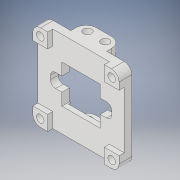
# Autodesk Inventor part: Camera_Cover
Saved by Autodesk Inventor 2019 (Build 230136000, 136)
## iProperties
Created: 2021-07-29
Part Number: Camera_Cover
Material: LCP 플라스틱
Document SubType Name: Modeling
Designer: user
Density: 1.626 g/cm^3
Appearance: 매끄러움 - 흰색
Mass: 4.96466 g
Surface Area: 31.5343 cm^2
Volume: 3.0533 cm^3
Author: user
Autodesk Inventor part; units mm, degrees
ref_plane "YZ Plane" through (0, 0, 0) normal (1, 0, 0) x (0, 1, 0)
ref_plane "XZ Plane" through (0, 0, 0) normal (0, 1, 0) x (-1, 0, 0)
ref_plane "XY Plane" through (0, 0, 0) normal (0, 0, 1) x (1, 0, 0)
sketch "스케치1" plane through (0, 0, 0) normal (0, 0, 1) x (1, 0, 0)
  line L0 (-16.9, 16.9) -> (16.9, 16.9)
  line L1 (16.9, 16.9) -> (16.9, -16.9)
  line L2 (16.9, -16.9) -> (-16.9, -16.9)
  line L3 (-16.9, -16.9) -> (-16.9, 16.9)
  point P0 (0, 0)
  dimension "d0" = 33.8
  dimension "d1" = 33.8
  dimension "d2" = 16.9
  dimension "d3" = 16.9
  constraints: 8 end point, 2 parallel, 1 horizontal, 1 perpendicular
  measures "d0" distance of L1.end L2.end
  measures "d1" distance of L0.end L1.end
  measures "d2" distance from line of L3 point (0, 0)
  measures "d3" distance from line of point (0, 0) L0
extrude "돌출1" add sketch "스케치1" along normal blind 3
sketch "스케치2" plane through (0, 0, 3) normal (0, 0, 1) x (1, 0, 0)
  circle A0 centre (-14, 14) radius 1.25
  circle A1 centre (14, 14) radius 1.25
  circle A2 centre (-14, -14) radius 1.25
  circle A3 centre (14, -14) radius 1.25
  line L0 (-16.9, 16.9) -> (-16.9, -16.9) projected
  line L1 (16.9, 16.9) -> (-16.9, 16.9) projected
  line L2 (16.9, -16.9) -> (16.9, 16.9) projected
  line L3 (-16.9, -16.9) -> (16.9, -16.9) projected
  line L4 (-16.9, 16.9) -> (-11.1, 16.9)
  line L5 (-11.1, 16.9) -> (-11.1, 11.1)
  line L6 (-11.1, 11.1) -> (-16.9, 11.1)
  line L7 (-16.9, 11.1) -> (-16.9, 16.9)
  line L8 (16.9, 16.9) -> (11.1, 16.9)
  line L9 (11.1, 16.9) -> (11.1, 11.1)
  line L10 (11.1, 11.1) -> (16.9, 11.1)
  line L11 (16.9, 11.1) -> (16.9, 16.9)
  line L12 (-16.9, -16.9) -> (-11.1, -16.9)
  line L13 (-11.1, -16.9) -> (-11.1, -11.1)
  line L14 (-11.1, -11.1) -> (-16.9, -11.1)
  line L15 (-16.9, -11.1) -> (-16.9, -16.9)
  line L16 (16.9, -16.9) -> (11.1, -16.9)
  line L17 (11.1, -16.9) -> (11.1, -11.1)
  line L18 (11.1, -11.1) -> (16.9, -11.1)
  line L19 (16.9, -11.1) -> (16.9, -16.9)
  point P0 (0, 0)
  dimension "d6" = 2.5
  dimension "d7" = 2.5
  dimension "d8" = 2.5
  dimension "d9" = 2.5
  dimension "d10" = 2.9
  dimension "d11" = 2.9
  dimension "d12" = 2.9
  dimension "d13" = 2.9
  dimension "d14" = 2.9
  dimension "d15" = 2.9
  dimension "d16" = 2.9
  dimension "d17" = 2.9
  dimension "d18" = 5.8
  dimension "d19" = 5.8
  dimension "d20" = 11.1
  dimension "d21" = 5.8
  dimension "d22" = 5.8
  dimension "d23" = 5.8
  dimension "d24" = 5.8
  dimension "d25" = 5.8
  dimension "d26" = 5.8
  constraints: 32 end point, 8 parallel, 4 centre point, 4 horizontal, 4 perpendicular
  measures "d6" diameter of A0
  measures "d7" diameter of A1
  measures "d8" diameter of A2
  measures "d9" diameter of A3
  measures "d10" distance from line of L0 A0.centre
  measures "d11" distance from line of L1 A0.centre
  measures "d12" distance from line of L2 A1.centre
  measures "d13" distance from line of L1 A1.centre
  measures "d14" distance from line of L3 A2.centre
  measures "d15" distance from line of L0 A2.centre
  measures "d16" distance from line of L3 A3.centre
  measures "d17" distance from line of L2 A3.centre
  measures "d18" distance of L5.end L6.end
  measures "d19" distance of L4.end L5.end
  measures "d20" distance from line of point (0, 0) L5
  measures "d21" distance of L10.end L9.end
  measures "d22" distance of L9.end L8.end
  measures "d23" distance of L14.end L13.end
  measures "d24" distance of L13.end L12.end
  measures "d25" distance of L17.end L18.end
  measures "d26" distance of L16.end L17.end
extrude "돌출2" add sketch "스케치2" along normal blind 2 contours A0 | A1 | A2 | A3 | L1 L5 L6 L0 | L14 L13 L3 L0 | L1 L2 L10 L9 | L17 L18 L2 L3
sketch "스케치3" plane through (0, 0, 5) normal (0, 0, 1) x (1, 0, 0)
  circle A0 centre (-14, 14) radius 1.5
  circle A1 centre (14, 14) radius 1.5
  circle A2 centre (14, -14) radius 1.5
  circle A3 centre (-14, -14) radius 1.5
  line L0 (-16.9, -11.1) -> (-16.9, -16.9) projected
  line L1 (-16.9, -16.9) -> (-11.1, -16.9) projected
  line L2 (11.1, -16.9) -> (16.9, -16.9) projected
  line L3 (16.9, -16.9) -> (16.9, -11.1) projected
  line L4 (11.1, 11.1) -> (16.9, 11.1) projected
  line L5 (16.9, 11.1) -> (16.9, 16.9) projected
  line L6 (-16.9, 16.9) -> (-16.9, 11.1) projected
  line L7 (-11.1, 16.9) -> (-16.9, 16.9) projected
  point P0 (0, 0)
  dimension "d29" = 3
  dimension "d30" = 3
  dimension "d31" = 3
  dimension "d32" = 3
  dimension "d33" = 2.9
  dimension "d34" = 2.9
  dimension "d35" = 2.9
  dimension "d36" = 2.9
  dimension "d37" = 2.9
  dimension "d38" = 2.9
  dimension "d39" = 2.9
  dimension "d40" = 2.9
  constraints: 4 centre point
  measures "d29" diameter of A0
  measures "d30" diameter of A1
  measures "d31" diameter of A2
  measures "d32" diameter of A3
  measures "d33" distance from line of L0 A3.centre
  measures "d34" distance from line of L1 A3.centre
  measures "d35" distance from line of L2 A2.centre
  measures "d36" distance from line of L3 A2.centre
  measures "d37" distance from line of L4 A1.centre
  measures "d38" distance from line of L5 A1.centre
  measures "d39" distance from line of L6 A0.centre
  measures "d40" distance from line of L7 A0.centre
extrude "돌출3" cut sketch "스케치3" against normal up to surface (5 mm away)
sketch "스케치4" plane through (0, 0, 3) normal (0, 0, 1) x (1, 0, 0)
  line L0 (-7.5, 7.5) -> (7.5, 7.5)
  line L1 (7.5, 7.5) -> (7.5, -7.5)
  line L2 (7.5, -7.5) -> (-7.5, -7.5)
  line L3 (-7.5, -7.5) -> (-7.5, 7.5)
  point P0 (0, 0)
  dimension "d43" = 15
  dimension "d44" = 15
  dimension "d45" = 7.5
  dimension "d46" = 7.5
  constraints: 8 end point, 2 parallel, 1 horizontal, 1 perpendicular
  measures "d43" distance of L1.end L2.end
  measures "d44" distance of L0.end L1.end
  measures "d45" distance from line of point (0, 0) L0
  measures "d46" distance from line of L3 point (0, 0)
extrude "돌출4" cut sketch "스케치4" against normal up to surface (3 mm away)
sketch "스케치5" plane through (0, 0, 3) normal (0, 0, 1) x (1, 0, 0)
  line L0 (-7.5, -2.75) -> (-12, -2.75)
  line L1 (-12, -2.75) -> (-12, 2.75)
  line L2 (-12, 2.75) -> (-7.5, 2.75)
  line L3 (-7.5, 2.75) -> (-7.5, -2.75)
  line L4 (7.5, 2.75) -> (12, 2.75)
  line L5 (12, 2.75) -> (12, -2.75)
  line L6 (12, -2.75) -> (7.5, -2.75)
  line L7 (7.5, -2.75) -> (7.5, 2.75)
  line L8 (-7.5, -7.5) -> (-7.5, 7.5) projected
  line L9 (7.5, 7.5) -> (7.5, -7.5) projected
  point P0 (0, 0)
  dimension "d49" = 4.5
  dimension "d50" = 5.5
  dimension "d51" = 4.5
  dimension "d52" = 5.5
  dimension "d53" = 0
  dimension "d54" = 2.75
  dimension "d55" = 0
  dimension "d56" = 2.75
  constraints: 16 end point, 4 parallel, 2 horizontal, 2 perpendicular
  measures "d49" distance of L1.end L2.end
  measures "d50" distance of L0.end L1.end
  measures "d51" distance of L5.end L6.end
  measures "d52" distance of L4.end L5.end
  measures "d53" distance between parallel lines of L8 L3
  measures "d54" distance from line of point (0, 0) L0
  measures "d55" distance between parallel lines of L9 L7
  measures "d56" distance from line of point (0, 0) L6
extrude "돌출5" cut sketch "스케치5" against normal up to surface (3 mm away)
fillet "모깎기1" radius 2 4 edges at (-12, 2.75, 1.5) (-12, -2.75, 1.5) (12, -2.75, 1.5) (12, 2.75, 1.5)
sketch "스케치6" plane through (0, 0, 0) normal (0, 0, -1) x (-1, 0, 0)
  line L0 (16.9, 16.9) -> (-16.9, 16.9) projected
  line L1 (-7, 16.9) -> (7, 16.9)
  line L2 (7, 16.9) -> (7, 12.9)
  line L3 (7, 12.9) -> (-7, 12.9)
  line L4 (-7, 12.9) -> (-7, 16.9)
  line L5 (-7, -16.9) -> (7, -16.9)
  line L6 (7, -16.9) -> (7, -12.9)
  line L7 (7, -12.9) -> (-7, -12.9)
  line L8 (-7, -12.9) -> (-7, -16.9)
  line L9 (-16.9, -16.9) -> (16.9, -16.9) projected
  point P0 (0, 0)
  dimension "d60" = 4
  dimension "d61" = 4
  dimension "d62" = 4
  dimension "d63" = 14
  dimension "d64" = 7
  dimension "d65" = 7
  dimension "d66" = 14
  constraints: 16 end point, 4 parallel, 2 horizontal, 2 perpendicular, 1 point on line
  measures "d60" distance between parallel lines of L7 L5
  measures "d61" distance between parallel lines of L9 L7
  measures "d62" distance between parallel lines of L3 L0
  measures "d63" distance between parallel lines of L2 L4
  measures "d64" distance from line of point (0, 0) L2
  measures "d65" distance from line of point (0, 0) L6
  measures "d66" distance between parallel lines of L6 L8
extrude "돌출6" add sketch "스케치6" along normal blind 6
sketch "스케치7" plane through (-11.1, -16.9, 3) normal (0, -1, 0) x (1, 0, 0)
  circle A0 centre (14.6, -6) radius 1.6
  circle A1 centre (7.6, -6) radius 1.6
  line L0 (18.1, -3) -> (18.1, -9) projected
  line L1 (4.1, -3) -> (4.1, -9) projected
  line L2 (18.1, -9) -> (4.1, -9) projected
  point P0 (11.1, -3)
  dimension "d69" = 3.2
  dimension "d70" = 3.5
  dimension "d71" = 3.5
  dimension "d72" = 3
  dimension "d73" = 3
  dimension "d74" = 3.2
  constraints: 2 centre point
  measures "d69" diameter of A1
  measures "d70" distance from line of L0 A0.centre
  measures "d71" distance from line of L1 A1.centre
  measures "d72" distance from line of L2 A0.centre
  measures "d73" distance from line of A1.centre L2
  measures "d74" diameter of A0
extrude "돌출7" cut sketch "스케치7" against normal up to surface (33.8 mm away)
fillet "모깎기2" radius 4 4 edges at (-7, 14.9, -6) (7, 14.9, -6) (-7, -14.9, -6) (7, -14.9, -6)
fillet "모깎기2" radius 3 4 edges at (-16.9, 16.9, 2.5) (-16.9, -16.9, 2.5) (16.9, 16.9, 2.5) (16.9, -16.9, 2.5)
sketch "스케치10" plane through (0, 0, 0) normal (0, 0, -1) x (-1, 0, 0)
  line L0 (7, -16.9) -> (7, -12.9) projected
  line L1 (-7.5, -7.5) -> (7.5, -7.5) projected
  line L2 (7, -12.9) -> (-7, -12.9)
  line L3 (-7, -12.9) -> (-7, -7.5)
  line L4 (-7, -7.5) -> (7, -7.5)
  line L5 (7, -7.5) -> (7, -12.9)
  line L6 (-7, -12.9) -> (-7, -16.9) projected
  line L7 (-7.5, 7.5) -> (7.5, 7.5) projected
  line L8 (-7, 12.9) -> (7, 12.9)
  line L9 (7, 12.9) -> (7, 7.5)
  line L10 (7, 7.5) -> (-7, 7.5)
  line L11 (-7, 7.5) -> (-7, 12.9)
  point P0 (0, 0)
  dimension "d94" = 14
  dimension "d96" = 14
  dimension "d99" = 14
  constraints: 16 end point, 4 parallel, 2 horizontal, 2 perpendicular, 2 point on line
  measures "d94" distance between parallel lines of L0 L6
  measures "d96" distance between parallel lines of L9 L11
  measures "d99" distance between parallel lines of L3 L5
extrude "돌출10" cut sketch "스케치10" against normal blind 1
equation "\"d2\" = 0.5 * d0"
equation "\"d3\" = 0.5 * d1"
equation "\"d45\" = 0.5 * d44"
equation "\"d46\" = 0.5 * d43"
equation "\"d54\" = 0.5 * d50"
equation "\"d56\" = 0.5 * d52"
equation "\"d64\" = 0.5 * d63"
equation "\"d65\" = 0.5 * d66"
equation "\"d72\" = d73"
equation "\"d96\" = d94"
